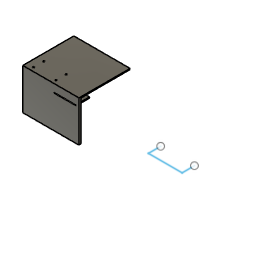
bedroom (Autodesk Fusion 360 design; units mm, degrees)
part number: 2025-06-26-09-06-35-783
Autodesk Fusion 360 part; units mm, degrees
sketch "Sketch1" plane through (0, 0, 0) normal (0, 0, 1) x (1, 0, 0)
  line L0 (-14, -13) -> (19, -13)
  line L1 (19, -13) -> (19, -1)
  line L2 (-14, -1) -> (-14, -13)
  constraint horizontal L0
  constraint vertical L1
  constraint vertical L2
sketch "Sketch2" plane through (0, 0, 0) normal (0, 0, 1) x (1, 0, 0)
  line L0 (4.5, -4.5) -> (-5.217, -4.5)
  line L1 (-5.217, -4.5) -> (-5.217, 0.8125)
  line L2 (-5.217, 0.8125) -> (4.5, 0.8125)
  line L3 (4.5, 0.8125) -> (4.5, -4.5)
  constraint horizontal L0
  constraint vertical L1
  constraint horizontal L2
  constraint vertical L3
extrude "Extrude1" add sketch "Sketch2" along normal blind 2 makes body 1
delete_face "DeleteFace1" 6 faces at (-1.978, 0.8125, 0.6667) (-1.978, -0.9583, 2) (-5.217, -2.7292, 0.6667) (-1.978, -0.9583, 0) (1.261, -4.5, 0.6667) (4.5, -0.9583, 0.6667) on bodies 1
sketch "Sketch3" plane through (0, 0, 0) normal (0, 0, 1) x (1, 0, 0)
  line L0 (0, 0) -> (100, 0)
  line L1 (100, 0) -> (100, 50.2805)
  line L2 (100, 50.2805) -> (0, 50.2805)
  line L3 (0, 50.2805) -> (0, 0)
  dimension "d3" = 100
  constraint horizontal L0
  constraint vertical L1
  constraint horizontal L2
  constraint vertical L3
  constraint coincident L0.start L3.end
  measures "d3" distance of L0.start L0.end
sketch "Sketch4" plane through (0, 0, 0) normal (0, 1, 0) x (1, 0, 0)
  line L0 (0, 0) -> (100, 0)
  line L1 (100, 0) -> (100, 40)
  line L2 (100, 40) -> (0, 40)
  line L3 (0, 40) -> (0, 0)
  constraint horizontal L0
  constraint vertical L1
  constraint horizontal L2
  constraint vertical L3
  constraint coincident L0.start L3.end
sketch "Sketch5" plane through (0, 0, 0) normal (0, 0, 1) x (1, 0, 0)
  line L0 (-50, 0) -> (-150, 0)
  line L1 (-150, 0) -> (-150, 50)
  line L2 (-150, 50) -> (-50, 50)
  line L3 (-50, 50) -> (-50, 0)
  constraint horizontal L0
  constraint vertical L1
  constraint horizontal L2
  constraint vertical L3
extrude "Extrude4" add sketch "Sketch5" against normal blind 40 separate body makes body 2
sketch "Sketch6" plane through (-50, 0, 0) normal (1, 0, 0) x (0, 1, 0)
  line L0 (50, 0) -> (0, 0)
  line L1 (0, 0) -> (0, -40)
  line L2 (0, -40) -> (50, -40)
  line L3 (50, -40) -> (50, 0)
  line L4 (50, -40) -> (2, -40)
  line L5 (2, -40) -> (2, -1)
  line L6 (2, -1) -> (50, -1)
  line L7 (50, -1) -> (50, -40)
  constraint horizontal L4
  constraint vertical L5
  constraint horizontal L6
  constraint vertical L7
  constraint coincident L2.end L3.start
extrude "Extrude5" cut sketch "Sketch6" against normal blind 95 contours L2 L3 L4 L5 L6 L7 bodies 2
sketch "Sketch7" plane through (0, 0, -1) normal (0, 0, -1) x (1, 0, 0)
  line L0 (-50, -50) -> (-50, -2)
  line L1 (-50, -2) -> (-145, -2)
  line L2 (-145, -2) -> (-145, -50)
  line L3 (-145, -50) -> (-50, -50)
sketch "Sketch8" plane through (0, 0, -1) normal (0, 0, -1) x (1, 0, 0)
  line L0 (-145, -2) -> (-120, -2)
  line L1 (-120, -2) -> (-120, -15)
  line L2 (-120, -15) -> (-145, -15)
  line L3 (-145, -15) -> (-145, -2)
  constraint horizontal L0
  constraint vertical L1
  constraint horizontal L2
  constraint vertical L3
extrude "Extrude6" add sketch "Sketch8" along normal blind 3 separate body makes body 3
move_body "Move1" bodies 3 to x (1, 0, 0) y (0, 1, 0) z (0, 0, 1) at (0, 0, -1)
sketch "Sketch9" plane through (0, 0, -5) normal (0, 0, -1) x (1, 0, 0)
  line L0 (-145, -15) -> (-120, -15)
  line L1 (-120, -15) -> (-120, -2)
  line L2 (-120, -2) -> (-145, -2)
  line L3 (-145, -2) -> (-145, -15)
  circle A0 centre (-121.25, -13.75) radius 0.7649
extrude "Extrude7" add sketch "Sketch9" along normal blind 2 separate body contours A0 makes body 4
pattern_linear "R-Pattern1" count 1 spacing 0 along (0, 1, 0) count 2 spacing 22 along (-1, 0, 0) of bodies 4 makes body 5
pattern_linear "R-Pattern2" count 2 spacing 10 along (0, -1, 0) of bodies 5 4 makes body 6 at (-121.1549, 2.9911, -6.3333) makes body 7 at (-142.5974, 3.3512, -6.3333)
move_body "Move2" bodies 7 5 6 4 to x (1, 0, 0) y (0, 1, 0) z (0, 0, 1) at (0, 0, 5)
sketch "Sketch10" plane through (0, 0, -5) normal (0, 0, -1) x (1, 0, 0)
  line L0 (-145, -15) -> (-120, -15)
  line L1 (-120, -15) -> (-120, -2)
  line L2 (-120, -2) -> (-145, -2)
  line L3 (-145, -2) -> (-145, -15)
  line L4 (-143, -5) -> (-140, -5)
  line L5 (-140, -5) -> (-140, -12)
  line L6 (-140, -12) -> (-143, -12)
  line L7 (-143, -12) -> (-143, -5)
  constraint horizontal L4
  constraint vertical L5
  constraint horizontal L6
  constraint vertical L7
extrude "Extrude8" add sketch "Sketch10" along normal blind 0.5 contours L4 L5 L6 L7 bodies 3
sketch "Sketch11" plane through (0, 0, -5) normal (0, 0, -1) x (1, 0, 0)
  line L0 (-143, -12) -> (-143, -5)
  line L1 (-143, -5) -> (-140, -5)
  line L2 (-140, -5) -> (-140, -12)
  line L3 (-140, -12) -> (-143, -12)
  line L4 (-145, -15) -> (-120, -15)
  line L5 (-120, -15) -> (-120, -2)
  line L6 (-120, -2) -> (-145, -2)
  line L7 (-145, -2) -> (-145, -15)
  line L8 (-139, -2) -> (-120, -2)
  line L9 (-120, -2) -> (-120, -15)
  line L10 (-120, -15) -> (-139, -15)
  line L11 (-139, -15) -> (-139, -2)
  constraint horizontal L8
  constraint vertical L9
  constraint horizontal L10
  constraint vertical L11
  constraint coincident L4.end L5.start
  constraint coincident L6 L8.start
extrude "Extrude9" add sketch "Sketch11" along normal blind 0.5 contours L4 L5 L6 L8 L9 L10 L11 bodies 2 4 5 6 7 3
sketch "Sketch12" plane through (0, 0, -1) normal (0, 0, -1) x (1, 0, 0)
  line L0 (-145, -20) -> (-137, -20)
  line L1 (-137, -20) -> (-137, -37)
  line L2 (-137, -37) -> (-145, -37)
  line L3 (-145, -37) -> (-145, -20)
  constraint horizontal L0
  constraint vertical L1
  constraint horizontal L2
  constraint vertical L3
extrude "Extrude10" add sketch "Sketch12" along normal blind 6 bodies 2
sketch "Sketch13" plane through (-137, 0, 0) normal (1, 0, 0) x (0, 1, 0)
  line L0 (37, -1) -> (20, -1)
  line L1 (20, -1) -> (20, -7)
  line L2 (20, -7) -> (37, -7)
  line L3 (37, -7) -> (37, -1)
  circle A0 centre (28.042, -4.0863) radius 1
extrude "Extrude11" add sketch "Sketch13" along normal blind 0.1 contours A0 bodies 2
sketch "Sketch14" plane through (0, 0, -1) normal (0, 0, -1) x (1, 0, 0)
  circle A0 centre (-110, -5) radius 1
extrude "Extrude12" add sketch "Sketch14" along normal blind 7 bodies 2
sketch "Sketch15" plane through (0, 0, -1) normal (0, 0, -1) x (1, 0, 0)
extrude "Extrude13" cut 1 faces at (-110.1218, 5.3103, -8) along direction (0, 0, 1) blind 7 on bodies 2 bodies 2
sketch "Sketch16" plane through (0, 0, -1) normal (0, 0, -1) x (1, 0, 0)
  circle A0 centre (-114, -6) radius 1
extrude "Extrude14" add sketch "Sketch16" along normal blind 7 separate body makes body 8
copy_body "CopyPasteBodies1" bodies 8 makes body 9
move_body "Move3" bodies 9 to x (1, 0, 0) y (0, 1, 0) z (0, 0, 1) at (12, 0, 0)
copy_body "CopyPasteBodies2" bodies 8 9 makes body 10 makes body 11
move_body "Move4" bodies 10 11 to x (1, 0, 0) y (0, 1, 0) z (0, 0, 1) at (0, 5, 0)
sketch "Sketch17" plane through (0, 0, -1) normal (0, 0, -1) x (1, 0, 0)
  line L0 (-118.4929, -1.8842) -> (-97, -1.8842)
  line L1 (-97, -1.8842) -> (-97, -15)
  line L2 (-97, -15) -> (-118.4929, -15)
  line L3 (-118.4929, -15) -> (-118.4929, -1.8842)
  constraint horizontal L0
  constraint vertical L1
  constraint horizontal L2
  constraint vertical L3
extrude "Extrude15" add sketch "Sketch17" along normal blind 1 separate body makes body 12
move_body "Move5" bodies 12 to x (1, 0, 0) y (0, 1, 0) z (0, 0, 1) at (-1.1479, -2.8593, -6.1392)
move_body "Move6" bodies 12 to x (1, 0, 0) y (0, 1, 0) z (0, 0, 1) at (0.0339, 1.3604, -0.314)
extrude "Extrude16" cut 1 faces at (-50, 0.6667, -13.6667) along direction (-1, 0, 0) blind 45 on bodies 2 bodies 2
sketch "Sketch18" plane through (0, 0, -1) normal (0, 0, -1) x (1, 0, 0)
  line L0 (-95, -50) -> (-95, -2)
  line L1 (-95, -2) -> (-145, -2)
  line L2 (-145, -2) -> (-145, -20)
  line L3 (-145, -20) -> (-137, -20)
  line L4 (-137, -20) -> (-137, -37)
  line L5 (-137, -37) -> (-145, -37)
  line L6 (-145, -37) -> (-145, -50)
  line L7 (-145, -50) -> (-95, -50)
  circle A0 centre (-112, -15) radius 1
extrude "Extrude17" add sketch "Sketch18" along normal blind 3 contours A0 bodies 2
delete_face "DeleteFace3" 1 faces at (-111.5887, 14.0885, -3) on bodies 2
sketch "Sketch19" plane through (0, 0, -1) normal (0, 0, -1) x (1, 0, 0)
  line L0 (-95, -50) -> (-95, -2)
  line L1 (-95, -2) -> (-145, -2)
  line L2 (-145, -2) -> (-145, -20)
  line L3 (-145, -20) -> (-137, -20)
  line L4 (-137, -20) -> (-137, -37)
  line L5 (-137, -37) -> (-145, -37)
  line L6 (-145, -37) -> (-145, -50)
  line L7 (-145, -50) -> (-95, -50)
  circle A0 centre (-113, -16) radius 1
extrude "Extrude18" add sketch "Sketch19" along normal blind 3 separate body contours A0 makes body 13
copy_body "CopyPasteBodies3" bodies 13 makes body 14
move_body "Move7" bodies 14 to x (1, 0, 0) y (0, 1, 0) z (0, 0, 1) at (7, 0, 0)
move_face "MoveFace1" to x (1, 0, 0) y (0, 1, 0) z (0, 0, 1) at (3, 0, 0) 1 faces at (-112.5887, 15.0885, -3) on bodies 13
copy_body "CopyPasteBodies4" bodies 13 14 makes body 15 makes body 16
move_body "Move8" bodies 15 16 to x (1, 0, 0) y (0, 1, 0) z (0, 0, 1) at (0, 3, 1)
move_body "Move9" bodies 15 16 to x (1, 0, 0) y (0, 1, 0) z (0, 0, 1) at (0, 0, -1)
sketch "Sketch20" plane through (0, 0, -1) normal (0, 0, -1) x (1, 0, 0)
  line L0 (-95, -50) -> (-95, -2)
  line L1 (-95, -2) -> (-145, -2)
  line L2 (-145, -2) -> (-145, -20)
  line L3 (-145, -20) -> (-137, -20)
  line L4 (-137, -20) -> (-137, -37)
  line L5 (-137, -37) -> (-145, -37)
  line L6 (-145, -37) -> (-145, -50)
  line L7 (-145, -50) -> (-95, -50)
  line L8 (-111, -15) -> (-105, -15)
  line L9 (-105, -15) -> (-105, -20)
  line L10 (-105, -20) -> (-111, -20)
  line L11 (-111, -20) -> (-111, -15)
  constraint horizontal L8
  constraint vertical L9
  constraint horizontal L10
  constraint vertical L11
extrude "Extrude19" cut sketch "Sketch20" along normal blind 0.5 contours L8 L9 L10 L11 bodies 13 14 15 16
sketch "Sketch21" plane through (0, 0, -1) normal (0, 0, -1) x (1, 0, 0)
  line L0 (-95, -50) -> (-95, -2)
  line L1 (-95, -2) -> (-145, -2)
  line L2 (-145, -2) -> (-145, -20)
  line L3 (-145, -20) -> (-137, -20)
  line L4 (-137, -20) -> (-137, -37)
  line L5 (-137, -37) -> (-145, -37)
  line L6 (-145, -37) -> (-145, -50)
  line L7 (-145, -50) -> (-95, -50)
  line L8 (-111, -15) -> (-105, -15)
  line L9 (-105, -15) -> (-105, -20)
  line L10 (-105, -20) -> (-111, -20)
  line L11 (-111, -20) -> (-111, -15)
  constraint horizontal L8
  constraint vertical L9
  constraint horizontal L10
  constraint vertical L11
extrude "Extrude20" add sketch "Sketch21" along normal blind 0.5 separate body contours L8 L9 L10 L11 makes body 17
move_body "Move10" bodies 17 to x (1, 0, 0) y (0, 1, 0) z (0, 0, 1) at (0, 0, -3)
copy_body "CopyPasteBodies5" bodies 17 makes body 18
move_body "Move11" bodies 18 to x (1, 0, 0) y (0, 0, -1) z (0, 1, 0) at (0, 24, 10.5)
named bodies: "bedleg", "bedleg (1)", "bedleg (2)", "bedleg (3)"
